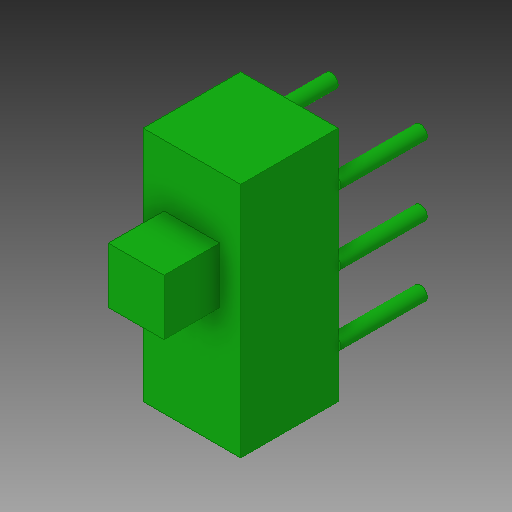
# Autodesk Inventor part: IS-1250
Saved by Autodesk Inventor 2018 (Build 220112000, 112)
## iProperties
Part Number: IS-1250
Material: 一般
Document SubType Name: Modeling
Designer: sktom
Density: 1 g/cm^3
Appearance: 濃い緑
Author: sktom
Autodesk Inventor part; units mm, degrees
ref_plane "YZ Plane" through (0, 0, 0) normal (1, 0, 0) x (0, 1, 0)
ref_plane "XZ Plane" through (0, 0, 0) normal (0, 1, 0) x (-1, 0, 0)
ref_plane "XY Plane" through (0, 0, 0) normal (0, 0, 1) x (1, 0, 0)
sketch "スケッチ1" plane through (0, 0, 0) normal (0, 0, 1) x (1, 0, 0)
  line L0 (-1.75, -4.25) -> (1.75, -4.25)
  line L1 (1.75, -4.25) -> (1.75, 4.25)
  line L2 (1.75, 4.25) -> (-1.75, 4.25)
  line L3 (-1.75, 4.25) -> (-1.75, -4.25)
  line L4 (-1.75, -4.25) -> (1.75, 4.25) construction
  line L5 (1.75, -4.25) -> (-1.75, 4.25) construction
  point P0 (0, 0)
  dimension "d0" = 3.5
  dimension "d1" = 8.5
  constraints: 12 end point, 2 midpoint, 2 parallel, 1 horizontal, 1 perpendicular
  measures "d0" distance of L1.end L2.end
  measures "d1" distance of L0.end L1.end
extrude "押し出し1" add sketch "スケッチ1" along normal blind 3.5
sketch "スケッチ2" plane through (0, 0, 0) normal (0, 0, -1) x (-1, 0, 0)
  line L0 (1.6, -2.5) -> (-1.6, -2.5) construction
  line L1 (-1.6, -2.5) -> (-1.6, 2.5) construction
  line L2 (-1.6, 2.5) -> (1.6, 2.5) construction
  line L3 (1.6, 2.5) -> (1.6, -2.5) construction
  line L4 (1.6, -2.5) -> (-1.6, 2.5) construction
  line L5 (-1.6, -2.5) -> (1.6, 2.5) construction
  circle A0 centre (-1.6, -2.5) radius 0.25
  point P0 (0, 0)
  dimension "d4" = 3.2
  dimension "d5" = 5
  dimension "d6" = 0.5
  constraints: 12 end point, 2 midpoint, 2 parallel, 1 centre point, 1 coincident, 1 horizontal, 1 perpendicular
  measures "d4" distance of L1.end L2.end
  measures "d5" distance of L0.end L1.end
  measures "d6" diameter of A0
extrude "押し出し2" add sketch "スケッチ2" along normal blind 3.1
pattern_linear "矩形状パターン1" count 3 spacing 2.5 along (0, 1, 0) count 2 spacing 3.2 along (-1, 0, 0) of "押し出し2"
sketch "スケッチ3" plane through (0, 0, 3.5) normal (0, 0, 1) x (1, 0, 0)
  line L0 (-1, 0.05) -> (1, 0.05)
  line L1 (1, 0.05) -> (1, 2.05)
  line L2 (1, 2.05) -> (-1, 2.05)
  line L3 (-1, 2.05) -> (-1, 0.05)
  line L4 (-1, 0.05) -> (1, 2.05) construction
  line L5 (1, 0.05) -> (-1, 2.05) construction
  line L6 (1.75, 4.25) -> (-1.75, 4.25) projected
  point P0 (0, 0)
  point P1 (0, 1.05)
  point P2 (0, 1.05)
  dimension "d15" = 2
  dimension "d16" = 4.2
  constraints: 12 end point, 3 midpoint, 2 parallel, 2 perpendicular, 1 horizontal, 1 vertical alignment
  measures "d15" distance of L2.end L0.start
  measures "d16" distance between parallel lines of L0 L6
extrude "押し出し3" add sketch "スケッチ3" along normal blind 2
